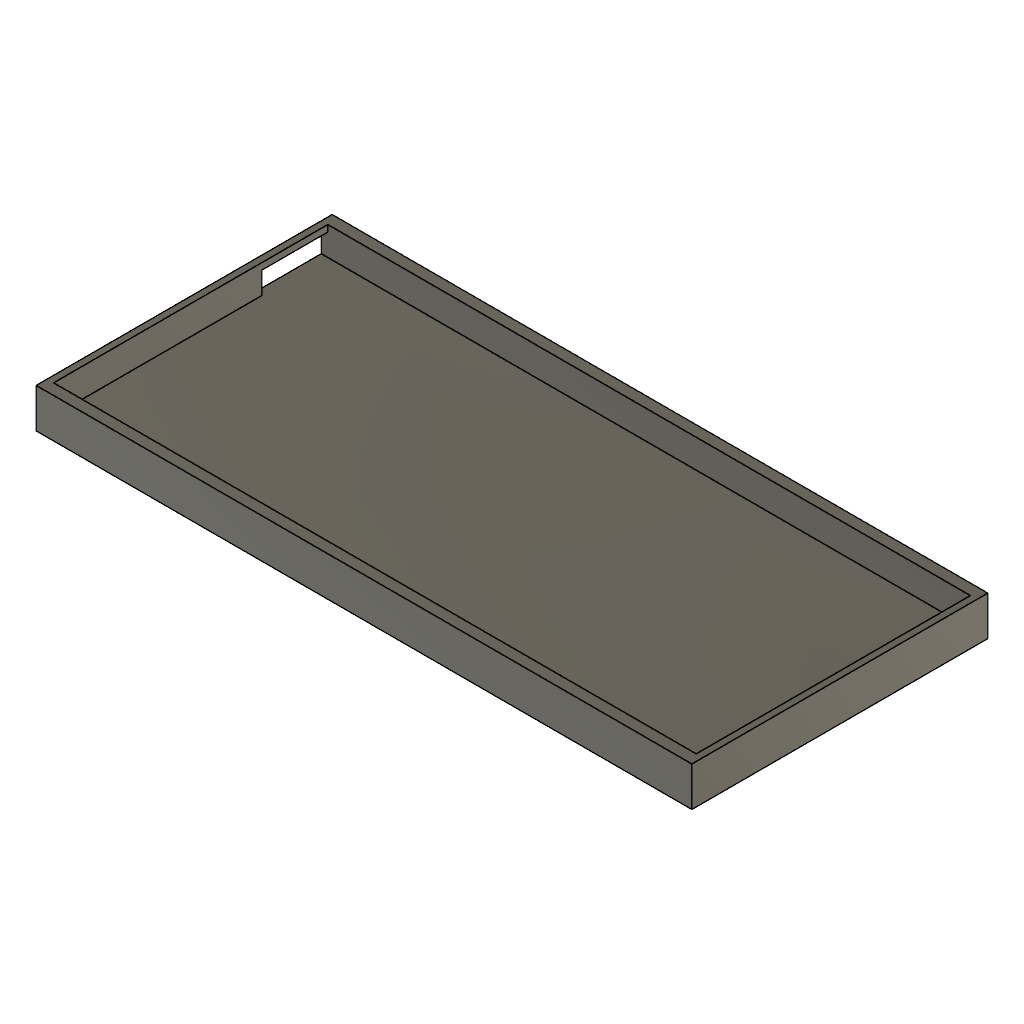
keyboatd (Autodesk Fusion 360 design; units mm, degrees)
part number: 2026-09-29-00-22-56-937
Autodesk Fusion 360 part; units mm, degrees
sketch "Sketch1" plane through (0, 0, 0) normal (0, 0, 1) x (1, 0, 0)
  line L0 (0, 0) -> (299, 0)
  line L1 (299, 0) -> (299, 135)
  line L2 (299, 135) -> (0, 135)
  line L3 (0, 135) -> (0, 0)
  line L4 (0, 135) -> (3, 135)
  line L5 (3, 130) -> (296, 130)
  line L6 (296, 130) -> (296, 5)
  line L7 (296, 5) -> (3, 5)
  line L8 (3, 5) -> (3, 130)
  dimension "d1" = 299
  dimension "d2" = 135
  dimension "d3" = 3
  constraint horizontal L0
  constraint vertical L1
  constraint horizontal L2
  constraint vertical L3
  constraint coincident L0.start L3.end
  constraint horizontal L4
  constraint horizontal L5
  constraint vertical L6
  constraint horizontal L7
  constraint vertical L8
  measures "d1" distance of L0.start L0.end
  measures "d2" distance of L0.start L2.end
  measures "d3" distance of L2.end L4.end
extrude "Extrude1" add sketch "Sketch1" along normal blind 13
sketch "Sketch2" plane through (0, 0, 0) normal (0, 0, 1) x (1, 0, 0)
  line L0 (3, 130) -> (296, 130)
  line L1 (296, 130) -> (296, 5)
  line L2 (296, 5) -> (3, 5)
  line L3 (3, 5) -> (3, 130)
  constraint horizontal L0
  constraint vertical L1
  constraint horizontal L2
  constraint vertical L3
extrude "Extrude2" add sketch "Sketch2" along normal blind 3
extrude "Extrude3" add 1 faces at (100.6667, 1.6667, 13) along direction (0, 0, 1) blind 5
extrude "Extrude4" add 1 faces at (100.6667, 88.3333, 3) along direction (0, 0, 1) blind 2
sketch "Sketch3" plane through (0, 0, 0) normal (-1, 0, 0) x (0, -1, 0)
  line L0 (-135, 0) -> (0, 0)
  line L1 (0, 0) -> (0, 18)
  line L2 (0, 18) -> (-135, 18)
  line L3 (-135, 18) -> (-135, 0)
  line L4 (-130, 15) -> (-100, 15)
  line L5 (-100, 15) -> (-100, 5)
  line L6 (-100, 5) -> (-130, 5)
  line L7 (-130, 5) -> (-130, 15)
  dimension "d12" = 10
  constraint horizontal L4
  constraint vertical L5
  constraint horizontal L6
  constraint vertical L7
  measures "d12" distance of L4.start L6.end
extrude "Extrude5" cut sketch "Sketch3" against normal blind 10 contours L4 L5 L6 L7
